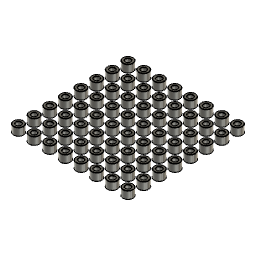
brusetniki-beads (Autodesk Fusion 360 design; units mm, degrees)
part number: 2025-08-05-22-05-54-821
Autodesk Fusion 360 part; units mm, degrees
sketch "Sketch1" plane through (0, 0, 0) normal (0, 0, 1) x (1, 0, 0)
  circle A0 centre (-3.0199, 3.0466) radius 3.2
  circle A1 centre (-3.0199, 3.0466) radius 1.6
  dimension "d1" = 6.4
  dimension "d2" = 3.2
  constraint concentric A0 A1
  measures "d1" diameter of A0
  measures "d2" diameter of A1
extrude "Extrude1" add sketch "Sketch1" along normal blind 5 makes body 1
fillet "Fillet1" radius 0.2 1 faces at (-0.3651, 2.8876, 5) on bodies 1
fillet "Fillet2" radius 0.2 1 faces at (-0.3651, 2.8876, 0) on bodies 1
move_body "Move1" bodies 1 to x (1, 0, 0) y (0, 1, 0) z (0, 0, 1) at (-2, 2, 0)
copy_body "CopyPasteBodies1" bodies 1 makes body 2
move_body "Move2" bodies 2 to x (1, 0, 0) y (0, 1, 0) z (0, 0, 1) at (-10, 0, 0)
copy_body "CopyPasteBodies2" bodies 2 makes body 3
move_body "Move3" bodies 3 to x (1, 0, 0) y (0, 1, 0) z (0, 0, 1) at (-10, 0, 0)
copy_body "CopyPasteBodies5" bodies 3 makes body 4
move_body "Move6" bodies 4 to x (1, 0, 0) y (0, 1, 0) z (0, 0, 1) at (-10, 0, 0)
copy_body "CopyPasteBodies6" bodies 4 makes body 5
move_body "Move7" bodies 5 to x (1, 0, 0) y (0, 1, 0) z (0, 0, 1) at (-10, 0, 0)
copy_body "CopyPasteBodies7" bodies 5 makes body 6
move_body "Move8" bodies 6 to x (1, 0, 0) y (0, 1, 0) z (0, 0, 1) at (-10, 0, 0)
copy_body "CopyPasteBodies8" bodies 6 makes body 7
move_body "Move9" bodies 7 to x (1, 0, 0) y (0, 1, 0) z (0, 0, 1) at (-10, 0, 0)
copy_body "CopyPasteBodies9" bodies 7 makes body 8
move_body "Move10" bodies 8 to x (1, 0, 0) y (0, 1, 0) z (0, 0, 1) at (-10, 0, 0)
copy_body "CopyPasteBodies10" bodies 1 2 3 4 5 6 7 8 makes body 9 makes body 10 makes body 11 makes body 12 makes body 13 makes body 14 makes body 15 makes body 16
move_body "Move11" bodies 9 10 11 12 13 14 15 16 to x (1, 0, 0) y (0, 1, 0) z (0, 0, 1) at (0, 10, 0)
copy_body "CopyPasteBodies11" bodies 9 10 11 12 13 14 15 16 makes body 17 makes body 18 makes body 19 makes body 20 makes body 21 makes body 22 makes body 23 makes body 24
move_body "Move12" bodies 17 18 19 20 21 22 23 24 to x (1, 0, 0) y (0, 1, 0) z (0, 0, 1) at (0, 10, 0)
copy_body "CopyPasteBodies12" bodies 17 18 19 20 21 22 23 24 makes body 25 makes body 26 makes body 27 makes body 28 makes body 29 makes body 30 makes body 31 makes body 32
move_body "Move13" bodies 25 26 27 28 29 30 31 32 to x (1, 0, 0) y (0, 1, 0) z (0, 0, 1) at (0, 10, 0)
copy_body "CopyPasteBodies13" bodies 25 26 27 28 29 30 31 32 makes body 33 makes body 34 makes body 35 makes body 36 makes body 37 makes body 38 makes body 39 makes body 40
move_body "Move14" bodies 33 34 35 36 37 38 39 40 to x (1, 0, 0) y (0, 1, 0) z (0, 0, 1) at (0, 10, 0)
copy_body "CopyPasteBodies14" bodies 33 34 35 36 37 38 39 40 makes body 41 makes body 42 makes body 43 makes body 44 makes body 45 makes body 46 makes body 47 makes body 48
move_body "Move15" bodies 41 42 43 44 45 46 47 48 to x (1, 0, 0) y (0, 1, 0) z (0, 0, 1) at (0, 10, 0)
copy_body "CopyPasteBodies15" bodies 41 42 43 44 45 46 47 48 makes body 49 makes body 50 makes body 51 makes body 52 makes body 53 makes body 54 makes body 55 makes body 56
move_body "Move16" bodies 49 50 51 52 53 54 55 56 to x (1, 0, 0) y (0, 1, 0) z (0, 0, 1) at (0, 10, 0)
copy_body "CopyPasteBodies16" bodies 49 50 51 52 53 54 55 56 makes body 57 makes body 58 makes body 59 makes body 60 makes body 61 makes body 62 makes body 63 makes body 64
move_body "Move17" bodies 57 58 59 60 61 62 63 64 to x (1, 0, 0) y (0, 1, 0) z (0, 0, 1) at (0, 10, 0)
named bodies: "Body4", "Body5", "Body6", "Body7", "Body7 (1)", "Body8", "Body4 (1)", "Body5 (1)", "Body6 (1)", "Body7 (2)", "Body8 (1)", "Body4 (1) (1)", "Body5 (1) (1)", "Body6 (1) (1)", "Body7 (2) (1)", "Body8 (1) (1)", "Body4 (1) (1) (1)", "Body5 (1) (1) (1)", "Body6 (1) (1) (1)", "Body7 (2) (1) (1)", "Body8 (1) (1) (1)", "Body4 (1) (1) (1) (1)", "Body5 (1) (1) (1) (1)", "Body6 (1) (1) (1) (1)", "Body7 (2) (1) (1) (1)", "Body8 (1) (1) (1) (1)", "Body4 (1) (1) (1) (1) (1)", "Body5 (1) (1) (1) (1) (1)", "Body6 (1) (1) (1) (1) (1)", "Body7 (2) (1) (1) (1) (1)", "Body8 (1) (1) (1) (1) (1)", "Body4 (1) (1) (1) (1) (1) (1)", "Body5 (1) (1) (1) (1) (1) (1)", "Body6 (1) (1) (1) (1) (1) (1)", "Body7 (2) (1) (1) (1) (1) (1)", "Body8 (1) (1) (1) (1) (1) (1)", "Body4 (1) (1) (1) (1) (1) (1) (1)", "Body5 (1) (1) (1) (1) (1) (1) (1)", "Body6 (1) (1) (1) (1) (1) (1) (1)", "Body7 (2) (1) (1) (1) (1) (1) (1)", "Body8 (1) (1) (1) (1) (1) (1) (1)"
